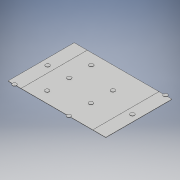
# Autodesk Inventor part: Croqui Vaso
Saved by Autodesk Inventor 2019 (Build 230136000, 136)
## iProperties
Created: 2018-12-02
Part Number: Croqui Vaso
Material: Generic
Document SubType Name: Modeling
Designer: leona
Density: 1 g/cm^3
Appearance: Default
Author: leona
Autodesk Inventor part; units mm, degrees
ref_plane "YZ Plane" through (0, 0, 0) normal (1, 0, 0) x (0, 1, 0)
ref_plane "XZ Plane" through (0, 0, 0) normal (0, 1, 0) x (-1, 0, 0)
ref_plane "XY Plane" through (0, 0, 0) normal (0, 0, 1) x (1, 0, 0)
sketch "Sketch1" plane through (0, 0, 0) normal (0, 1, 0) x (-1, 0, 0)
  line L0 (0, 0) -> (2700, 0)
  line L1 (2700, 0) -> (2700, -2492)
  line L2 (2700, -2492) -> (0, -2492)
  line L3 (0, -2492) -> (0, 0)
  dimension "d0" = 2700
  dimension "d1" = 2492
  constraints: 8 end point, 2 parallel, 1 horizontal, 1 perpendicular
  measures "d0" distance of L0.start L0.end
  measures "d1" distance of L0.end L1.end
extrude "Extrusion1" add sketch "Sketch1" along normal blind 10
sketch "Sketch2" plane through (0, 10, 0) normal (0, 1, 0) x (1, 0, 0)
  line L0 (-2700, 2492) -> (-2700, 0) projected
  line L1 (-2700, 0) -> (-3190, 0)
  line L2 (-3190, 0) -> (-3190, 2492)
  line L3 (-3190, 2492) -> (-2700, 2492)
  line L4 (-2700, 2492) -> (-2700, 0)
  line L5 (0, 2492) -> (-2700, 2492) projected
  line L6 (0, 0) -> (0, 2492) projected
  line L7 (0, 2492) -> (490, 2492)
  line L8 (490, 2492) -> (490, 0)
  line L9 (490, 0) -> (0, 0)
  line L10 (0, 0) -> (0, 2492)
  line L11 (-2700, 0) -> (0, 0) projected
  dimension "d4" = 490
  constraints: 16 end point, 4 parallel, 3 collinear, 2 horizontal, 2 perpendicular
  measures "d4" distance of L2.end L3.end
extrude "Extrusion2" add sketch "Sketch2" against normal blind 10 separate body
sketch "Sketch3" plane through (0, 10, 0) normal (0, 1, 0) x (1, 0, 0)
  circle A0 centre (245, 1246) radius 75
  line L0 (-3190, 2492) -> (490, 2492) projected
  circle A1 centre (245, 2492) radius 75
  circle A2 centre (-900, 0) radius 75
  circle A3 centre (-900, 830) radius 75
  circle A4 centre (-900, 1660) radius 75
  circle A5 centre (-2130, 415) radius 75
  circle A6 centre (-2130, 1245) radius 75
  circle A7 centre (-2130, 2075) radius 75
  circle A8 centre (-2945, 0) radius 75
  circle A9 centre (-2945, 1246) radius 75
  line L1 (0, 0) -> (0, 2492) projected
  line L2 (-3190, 0) -> (490, 0) projected
  line L3 (-2700, 2492) -> (-2700, 0) projected
  dimension "d7" = 150
  dimension "d8" = 900
  dimension "d9" = 2130
  dimension "d10" = 830
  dimension "d11" = 830
  dimension "d12" = 415
  dimension "d13" = 830
  dimension "d14" = 830
  dimension "d15" = 1246
  dimension "d16" = 245
  dimension "d17" = 245
  constraints: 10 centre point, 9 equal radius, 6 vertical alignment, 3 point on line, 1 horizontal alignment
  measures "d7" diameter of A9
  measures "d8" distance from line of L1 A4.centre
  measures "d9" distance from line of L1 A7.centre
  measures "d10" distance of A3.centre A2.centre
  measures "d11" distance of A4.centre A3.centre
  measures "d12" distance from line of L2 A5.centre
  measures "d13" distance of A6.centre A5.centre
  measures "d14" distance of A7.centre A6.centre
  measures "d15" distance from line of L2 A0.centre
  measures "d16" distance from line of L1 A1.centre
  measures "d17" distance from line of L3 A8.centre
extrude "Extrusion3" add sketch "Sketch3" along normal blind 10 contours A0 | A1 L0 | L0 A1 | A8 L2 | L2 A8 | L2 A2 | A2 L2 | A3 | A4 | A5 | A6 | A7 | A9 bodies 1
body "Solid1"
body "Solid2"
